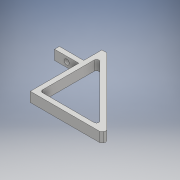
# Autodesk Inventor part: holder-LCD-v2
Saved by Autodesk Inventor 2018 (Build 220112000, 112)
## iProperties
Created: 2018-01-28
Part Number: holder-LCD-v2
Material: Generic
Document SubType Name: Modeling
Designer: Jurjen
Density: 1 g/cm^3
Appearance: Default
Author: Jurjen
Autodesk Inventor part; units mm, degrees
ref_plane "YZ Plane" through (0, 0, 0) normal (1, 0, 0) x (0, 1, 0)
ref_plane "XZ Plane" through (0, 0, 0) normal (0, 1, 0) x (-1, 0, 0)
ref_plane "XY Plane" through (0, 0, 0) normal (0, 0, 1) x (1, 0, 0)
sketch "Sketch1" plane through (0, 0, 0) normal (0, 0, 1) x (1, 0, 0)
  line L0 (-27.5, 24.6716) -> (21.8431, -24.6716)
  line L1 (31.5, -28.6716) -> (-27.5, 30.3284)
  line L2 (-27.5, 30.3284) -> (-31.5, 30.3284)
  line L3 (31.5, -28.6716) -> (-31.5, -28.6716)
  line L4 (-27.5, -24.6716) -> (21.8431, -24.6716)
  line L5 (-27.5, 24.6716) -> (-27.5, -24.6716)
  line L6 (-31.5, 15.3284) -> (-51.5, 15.3284)
  line L7 (-51.5, 15.3284) -> (-51.5, 11.3284)
  line L8 (-51.5, 11.3284) -> (-31.5, 11.3284)
  line L9 (-31.5, 30.3284) -> (-31.5, 15.3284)
  line L10 (-31.5, 11.3284) -> (-31.5, -28.6716)
  point P0 (0, 0)
  point P1 (-27.5, 0)
  point P2 (0, -28.6716)
  dimension "d0" = 4
  dimension "d19" = 4
  dimension "d22" = 20
  dimension "d23" = 4
  dimension "d25" = 45
  dimension "d28" = 83.4386
  dimension "d29" = 4
  dimension "d30" = 4
  dimension "d35" = 40
  constraints: 22 end point, 3 horizontal, 3 perpendicular, 2 midpoint, 2 vertical alignment, 1 horizontal alignment, 1 vertical
  measures "d0" distance between parallel lines of L1 L0
  measures "d19" distance between parallel lines of L3 L4
  measures "d22" distance of L6.end L6.start
  measures "d23" distance between parallel lines of L8 L6
  measures "d25" angle of L0 L5
  measures "d28" distance of L1.start L1.end
  measures "d29" distance between parallel lines of L5 L10
  measures "d30" distance of L2.end L1.end
  measures "d35" distance between parallel lines of L3 L8
extrude "Extrusion1" add sketch "Sketch1" along normal mid plane 8
sketch "Sketch5" plane through (-51.5, 15.3284, -4) normal (0, 1, 0) x (1, 0, 0)
  line L0 (20, -8) -> (20, 0) projected
  line L1 (0, 0) -> (20, 0) projected
  line L2 (0, -8) -> (0, 0) projected
  line L3 (20, -8) -> (0, -8) projected
  circle A0 centre (10, -4) radius 2.1
  point P0 (51.5, -4)
  point P1 (0, -4)
  dimension "d31" = 4.2
  dimension "d32" = 10
  constraints: 1 centre point, 1 horizontal alignment, 1 midpoint
  measures "d31" diameter of A0
  measures "d32" distance from line of A0.centre L2
extrude "Extrusion4" cut sketch "Sketch5" against normal through all contours A0
sketch "Sketch6" plane through (-27.5, 30.3284, -4) normal (0.7071, 0.7071, 0) x (-0.7071, 0.7071, 0)
  circle A0 centre (-13.9386, 4) radius 1.6
  circle A1 centre (-63.4386, 4) radius 1.6
  line L0 (-83.4386, 0) -> (-83.4386, 8) projected
  point P0 (-40.8909, 4)
  point P1 (-83.4386, 4)
  dimension "d36" = 49.5
  dimension "d37" = 20
  dimension "d38" = 3.2
  constraints: 2 centre point, 2 horizontal alignment, 1 equal radius, 1 midpoint
  measures "d36" distance of A1.centre A0.centre
  measures "d37" distance from line of A1.centre L0
  measures "d38" diameter of A1
extrude "Extrusion5" cut sketch "Sketch6" against normal blind 6
sketch "Sketch7" plane through (0, 0, 4) normal (0, 0, 1) x (1, 0, 0)
  line L0 (31.5, -28.6716) -> (-27.5, 30.3284) projected
  line L1 (-31.5, -28.6716) -> (31.5, -28.6716) projected
  line L2 (28.6716, -25.8431) -> (25.8431, -28.6716)
  line L3 (25.8431, -28.6716) -> (31.5, -28.6716)
  line L4 (28.6716, -25.8431) -> (31.5, -28.6716)
  point P0 (0, 0)
  dimension "d42" = 4
  constraints: 6 end point, 2 point on line, 1 horizontal, 1 perpendicular
  measures "d42" distance of L2.start L2.end
extrude "Extrusion6" cut sketch "Sketch7" against normal through all
fillet "Fillet1" radius 2 5 edges at (-27.5, -24.6716, 0) (-27.5, 30.3284, 0) (28.6716, -25.8431, 0) (21.8431, -24.6716, 0) (-27.5, 24.6716, 0)
body "Solid1"
